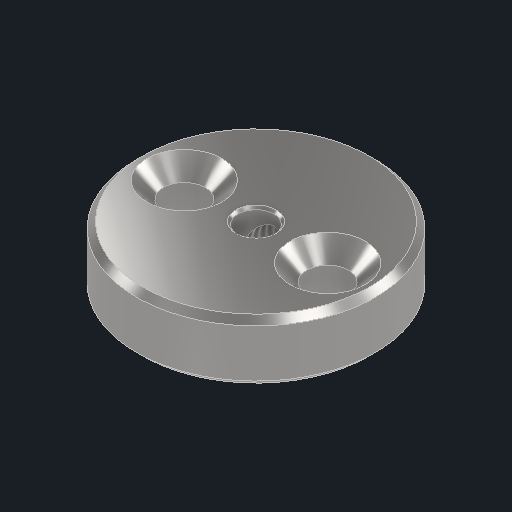
# Autodesk Inventor part: Wheel Mounting Cap
Saved by Autodesk Inventor 2027.1 (Build 311270010, 270A)
## iProperties
Created: 2025-09-16
Material: Mild Steel S355 J2
Document SubType Name: Modeling
Designer: SD
Density: 7.85 g/cm^3
Appearance: Semi-Polished
Mass: 10.4609 g
Surface Area: 10.6836 cm^2
Volume: 1.3326 cm^3
Project: Automatic Tea Steeping mechanism
Part Number: Wheel Mounting Cap
BOM-Mass: 0.01046
BOM-Area: 0.001
Diameter: 20.000 mm
Thickness: 5.000 mm
Procurement: Fabricate - 1st round
Build Stage: 2
Preferred Material: TBD
Author: SD
Title: Wheel Mounting Cap
Autodesk Inventor part; units mm, degrees
ref_plane "YZ Plane" through (0, 0, 0) normal (1, 0, 0) x (0, 1, 0)
ref_plane "XZ Plane" through (0, 0, 0) normal (0, 1, 0) x (-1, 0, 0)
ref_plane "XY Plane" through (0, 0, 0) normal (0, 0, 1) x (1, 0, 0)
sketch "Sketch4" plane through (0, 0, 0) normal (0, 1, 0) x (-1, 0, 0)
  circle A0 centre (0, 0) radius 10
  constraints: 1 centre point, 1 coincident, 1 other
extrude "Extrusion2" add sketch "Sketch4" along normal mid plane 5
sketch "Sketch8" plane through (0, 2.5, 0) normal (0, 1, 0) x (1, 0, 0)
  point P0 (0, 0)
  point P1 (-6, 0)
  point P2 (6, 0)
  dimension "d63" = 6
  dimension "d64" = 12
  constraints: 2 horizontal alignment
  measures "d63" distance of point (6, 0) point (0, 0)
  measures "d64" distance of point (-6, 0) point (6, 0)
hole "Hole5" at (-6, 2.5, 0) at (6, 2.5, 0) direction (0, -1, 0) diameter 3.5 depth 22.2 countersink diameter 6.3 countersink angle 90
sketch "Sketch9" plane through (0, 2.5, 0) normal (0, 1, 0) x (1, 0, 0)
  line L0 (-1.5, 1.5) -> (1.5, 1.5) construction
  line L1 (1.5, 1.5) -> (1.5, -1.5) construction
  line L2 (1.5, -1.5) -> (-1.5, -1.5) construction
  line L3 (-1.5, -1.5) -> (-1.5, 1.5) construction
  line L4 (-1.5, 1.5) -> (1.5, -1.5) construction
  line L5 (1.5, 1.5) -> (-1.5, -1.5) construction
  circle A0 centre (0, 0) radius 1.5
  dimension "d72" = 3
  dimension "d73" = 3
  dimension "d86" = 3
  constraints: 12 end point, 2 midpoint, 2 parallel, 1 centre point, 1 coincident, 1 horizontal, 1 perpendicular
  measures "d72" distance of L0.start L0.end
  measures "d73" distance of L0.end L1.end
  measures "d86" diameter of A0
extrude "Extrusion5" cut sketch "Sketch9" against normal blind 10
sketch "Sketch10" plane through (-1.5, 2.5, 0) normal (0, 0, 1) x (1, 0, 0)
  point P0 (1.5, -2.5)
  point P1 (1.5, -2.5)
  constraints: 1 coincident
hole "Hole6" at (0, 0, 0) direction (0, 0, -1) diameter 2.85 depth 10.4 thread size "M3.5x0.6" class "6H" standard "ISO Metric profile"
chamfer "Chamfer1" distance 0.5 angle 45 2 edges at (10, 2.5, 0) (10, -2.5, 0)
chamfer "Chamfer2" distance 0.2 angle 45 2 edges at (-1.5, 2.5, 0) (-1.5, -2.5, 0)
equation "\"d73\" = d72"
body "Solid2"
